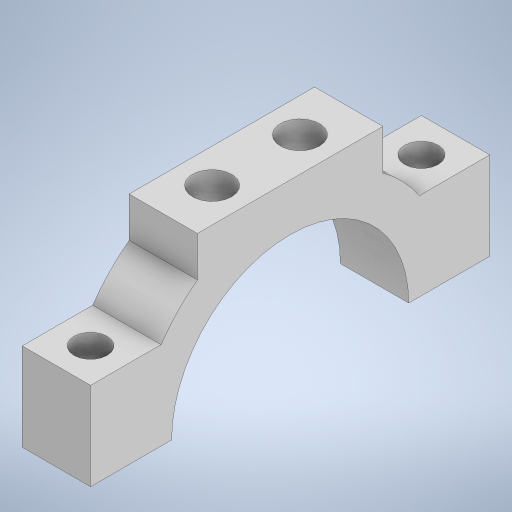
# Autodesk Inventor part: Motorhalter
Saved by Autodesk Inventor 2023 (Build 270158000, 158)
## iProperties
Created: 2023-03-30
Part Number: Motorhalter
Material: Generisch
Document SubType Name: Modeling
Designer: prigge
Density: 1 g/cm^3
Appearance: Vorgabe
Author: prigge
Autodesk Inventor part; units mm, degrees
ref_plane "YZ Plane" through (0, 0, 0) normal (1, 0, 0) x (0, 1, 0)
ref_plane "XZ Plane" through (0, 0, 0) normal (0, 1, 0) x (-1, 0, 0)
ref_plane "XY Plane" through (0, 0, 0) normal (0, 0, 1) x (1, 0, 0)
sketch "Skizze1" plane through (0, 0, 0) normal (1, 0, 0) x (0, 1, 0)
  circle A0 centre (0, 0) radius 12.15
  line L0 (0, 16.95) -> (23.4061, 16.95) construction
  line L1 (0, 20.45) -> (9, 20.45)
  arc A1 (16, 0) -> (9, 13.2288) centre (0, 0) ccw
  line L2 (9, 13.2288) -> (9, 20.45)
  line L3 (0, 20.45) -> (0, 12.15)
  line L4 (0, 28.63) -> (0, -28.63) projected
  line L5 (0, 0) -> (16, 0)
  line L6 (0, -20.45) -> (9, -20.45)
  arc A2 (9, -13.2288) -> (16, 0) centre (0, 0) ccw
  line L7 (9, -13.2288) -> (9, -20.45)
  line L8 (0, -20.45) -> (0, -12.15)
  point P0 (0, -12.15)
  dimension "d0" = 24.3
  dimension "d1" = 16.95
  dimension "d2" = 20.45
  dimension "d3" = 9
  dimension "d4" = 16
  constraints: 16 end point, 4 point on circle, 4 symmetric about line, 3 horizontal, 2 centre point, 2 coincident, 2 vertical, 1 point on line, 4 other
  measures "d1" distance from line of point (0, 0) L0
  measures "d2" distance from line of point (0, 0) L1
  measures "d3" distance between parallel lines of L3 L2
  measures "d4" radius of A1
extrude "Extrusion1" add sketch "Skizze1" against normal blind 7 contours L5 A2 L7 L6 L4 A0 | A0 L3 L1 L2 A1 L5
sketch "Skizze2" plane through (0, 0, 0) normal (0, 1, 0) x (-1, 0, 0)
  circle A0 centre (3.5, 16.95) radius 1.7
  circle A1 centre (3.5, -16.95) radius 1.7162
  line L0 (0, 20.45) -> (7, 20.45) projected
  line L1 (-1.4, 0) -> (8.4, 0) projected
  point P0 (0, 0)
  point P1 (3.5, 20.45)
  point P2 (3.5, 20.45)
  dimension "d9" = 33.9
  dimension "d10" = 3.4
  constraints: 2 centre point, 2 midpoint, 2 vertical alignment
  measures "d9" distance of A0.centre A1.centre
  measures "d10" diameter of A0
extrude "Extrusion2" cut sketch "Skizze2" along normal through all
sketch "Skizze3" plane through (0, 0, 0) normal (1, 0, 0) x (0, 1, 0)
  arc A0 (9, -13.2288) -> (9, 13.2288) centre (0, 0) ccw projected
  arc A1 (9, -13.2288) -> (9, 13.2288) centre (0, 0) ccw projected
  line L0 (17, 9.5) -> (12.8744, 9.5)
  line L1 (12.8744, 9.5) -> (12.8744, -9.5)
  line L2 (12.8744, -9.5) -> (17, -9.5)
  line L3 (17, -9.5) -> (17, 9.5)
  line L4 (0, -12.15) -> (0, -20.45) projected
  point P0 (12.8744, -9.5)
  dimension "d14" = 19
  dimension "d22" = 17
  constraints: 8 end point, 2 parallel, 2 point on circle, 1 horizontal, 1 perpendicular
  measures "d14" distance of L2.end L0.start
  measures "d22" distance between parallel lines of L4 L3
extrude "Extrusion3" add sketch "Skizze3" against normal up to surface (7 mm away) contours A0 L0 L3 L2
sketch "Skizze4" plane through (0, 17, 9.5) normal (0, 1, 0) x (1, 0, 0)
  circle A0 centre (-3.5, 5) radius 2
  circle A1 centre (-3.5, 14) radius 2
  line L0 (0, 9.5) -> (-10.2525, 9.5)
  line L1 (0, 19) -> (-7, 19) projected
  point P0 (-3.5, 19)
  dimension "d17" = 4
  dimension "d18" = 9
  constraints: 2 centre point, 2 end point, 2 vertical alignment, 1 equal radius, 1 horizontal, 1 midpoint, 1 symmetric about line
  measures "d17" diameter of A0
  measures "d18" distance of A1.centre A0.centre
extrude "Extrusion4" cut sketch "Skizze4" against normal blind 4
